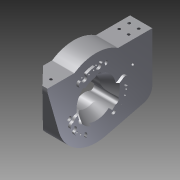
# Autodesk Inventor part: launcher.housing2
Saved by Autodesk Inventor 2011 (Build 150239000, 239)
## iProperties
Created: 2011-01-27
Part Number: launcher.housing2
Document SubType Name: Modeling
Designer: Casey
Density: 1 g/cm^3
Mass: 704.398 g
Surface Area: 699.987 cm^2
Volume: 704.398 cm^3
Author: Casey
Autodesk Inventor part; units mm, degrees
ref_plane "YZ Plane" through (0, 0, 0) normal (1, 0, 0) x (0, 1, 0)
ref_plane "XZ Plane" through (0, 0, 0) normal (0, 1, 0) x (-1, 0, 0)
ref_plane "XY Plane" through (0, 0, 0) normal (0, 0, 1) x (1, 0, 0)
sketch "Sketch1" plane through (0, 0, 0) normal (0, 0, 1) x (1, 0, 0)
  line L0 (2.019581, 25) -> (20, 35.381)
  line L1 (20, 35.381) -> (20, 70)
  line L2 (20, 70) -> (0, 70)
  line L3 (0, 0) -> (46.562095, 0) construction
  line L4 (0, 70) -> (0, 25)
  line L5 (0, 25) -> (2.019581, 25)
  line L6 (0, 25) -> (-20, 25)
  line L7 (-20, 25) -> (-20, 70)
  line L8 (-20, 70) -> (0, 70)
  dimension "d3" = 70
  dimension "d6" = 30
  dimension "d8" = 25
  dimension "d86" = 35.381
  dimension "d182" = 20
  dimension "d230" = 20
  constraints: 18 end point, 2 horizontal, 2 perpendicular, 2 vertical, 1 collinear, 1 parallel, 1 point on line, 1 other
  measures "d3" distance from line of L3.start L2
  measures "d6" angle of L5 L0
  measures "d8" distance from line of L3.start L5
  measures "d86" distance from line of L3 L0.end
  measures "d182" distance between parallel lines of L4 L1
  measures "d230" distance of L4.end L6.end
revolve "Revolution1" add sketch "Sketch1" angle 360 about axis through (0, 0, 0) along (1, 0, 0)
sketch "Sketch11" plane through (20, 0, 0) normal (1, 0, 0) x (0, 0, -1)
  circle A0 centre (0, 0) radius 35.381 projected
  line L0 (-35, -6) -> (0, -6)
  line L1 (0, -6) -> (0, 6)
  line L2 (0, 6) -> (-35, 6)
  arc A1 (-35, 6) -> (-35, -6) centre (-35, 0) ccw
  line L3 (-35, 0) -> (0, 0) construction
  dimension "d87" = 12
  dimension "d88" = 35
  constraints: 8 end point, 2 horizontal, 2 midpoint, 2 point on circle, 1 centre point, 1 parallel, 1 perpendicular, 1 point on line, 1 tangent
  measures "d87" diameter of A1
  measures "d88" distance of A0.centre L3.start
extrude "Extrusion10" cut sketch "Sketch11" against normal through all contours L2 L1 L0 A0 | A0 L0 A1 L2 picked at (-11.774646, -0.669544)
fillet "Fillet12" radius 20 2 edges at (-8.9902, 6, 24.2693) (-8.9902, -6, 24.2693)
pattern_circular "Circular Pattern6" count 3 over 360 about axis through (11.00979, 0, 0) along (1, 0, 0) of "Extrusion10", "Fillet12"
sketch "Sketch26" plane through (20, 0, 0) normal (1, 0, 0) x (0, 0, -1)
  arc A0 (12.208765, 33.207849) -> (12.520317, 33.657942) centre (-4.078625, 44.814783) ccw
  arc A1 (22.888474, 27.671884) -> (12.520317, 33.657942) centre (17.5, 30.310889) ccw
  arc A2 (22.888474, 27.671884) -> (22.654458, 27.177025) centre (40.850053, 18.875199) ccw
  arc A3 (22.654458, -27.177025) -> (22.654458, 27.177025) centre (0, 0) ccw
  arc A4 (22.654458, -27.177025) -> (22.888474, -27.671884) centre (40.850053, -18.875199) ccw
  arc A5 (12.520317, -33.657942) -> (22.888474, -27.671884) centre (17.5, -30.310889) ccw
  arc A6 (12.520317, -33.657942) -> (12.208765, -33.207849) centre (-4.078625, -44.814783) ccw
  arc A7 (-34.863223, -6.030824) -> (12.208765, -33.207849) centre (0, 0) ccw
  arc A8 (-34.863223, -6.030824) -> (-35.408791, -5.986058) centre (-36.771429, -25.939584) ccw
  arc A9 (-35.408791, 5.986058) -> (-35.408791, -5.986058) centre (-35, 0) ccw
  arc A10 (-35.408791, 5.986058) -> (-34.863223, 6.030824) centre (-36.771429, 25.939584) ccw
  arc A11 (12.208765, 33.207849) -> (-34.863223, 6.030824) centre (0, 0) ccw
  circle A12 centre (0, 0) radius 70
  circle A13 centre (0, 0) radius 54.5
  dimension "d183" = 109
  constraints: 1 centre point, 1 coincident
  measures "d183" diameter of A13
extrude "Extrusion14" add sketch "Sketch26" along normal blind 4.5 contours A13
sketch "Sketch27" plane through (0, 0, 0) normal (0, 0, 1) x (1, 0, 0)
  line L0 (20, 35.381) -> (24.5, 37.979076)
  line L1 (24.5, 37.979076) -> (24.5, 35.381)
  line L2 (24.5, 35.381) -> (20, 35.381)
  line L3 (20, 35.381) -> (2.42675, 25.235079)
  line L4 (24.5, 54.5) -> (24.5, -54.5)
  line L5 (0, 0) -> (24.5, 0) construction
  constraints: 8 end point, 2 collinear, 1 midpoint, 1 perpendicular, 1 vertical
revolve "Revolution3" cut sketch "Sketch27" angle 360 about axis through (0, 0, 0) along (1, 0, 0)
sketch "Sketch28" plane through (24.5, 0, 0) normal (1, 0, 0) x (0, 0, -1)
  arc A0 (23.482236, -29.849536) -> (23.482236, 29.849536) centre (0, 0) ccw
  arc A1 (14.109338, 35.260981) -> (-37.591575, 5.411445) centre (0, 0) ccw
  circle A2 centre (0, 0) radius 54.5 construction
  arc A3 (-51.213248, 18.640098) -> (-43.045959, 12.148551) centre (-46.044938, 16.758987) ccw
  circle A4 centre (-46.044938, 16.758987) radius 4 construction
  line L0 (0, 0) -> (-46.044938, 16.758987) construction
  line L1 (0, 0) -> (-54.5, 0) construction
  arc A5 (-35.688658, 12.989609) -> (-43.045959, 12.148551) centre (-38.52465, 5.197784) ccw
  line L2 (0, 0) -> (-27.25, 47.198385) construction
  line L3 (0, 0) -> (-41.749422, 35.031925) construction
  line L4 (0, 0) -> (-9.463826, 53.672023) construction
  arc A6 (-6.594997, 37.402089) -> (-18.086825, 51.411251) centre (-46.044938, 16.758987) ccw
  arc A7 (-18.086825, 51.411251) -> (-51.213248, 18.640098) centre (0, 0) ccw
  line L5 (-35.688658, 12.989609) -> (0, 0)
  line L6 (0, 0) -> (-1.913763, 10.853491)
  arc A8 (-1.913763, 10.853491) -> (-6.594997, 37.402089) centre (-46.044938, 16.758987) ccw
  dimension "d187" = 11
  dimension "d188" = 8
  dimension "d190" = 20
  dimension "d191" = 60
  dimension "d192" = 20
  constraints: 18 point on circle, 14 end point, 6 centre point, 5 point on line, 4 tangent, 3 coincident, 2 collinear, 2 concentric, 1 horizontal, 1 other
  measures "d187" diameter of A3
  measures "d188" diameter of A4
  measures "d190" angle of L1 L0
  measures "d191" angle of L1 L2
  measures "d192" angle of L2 L3
extrude "Extrusion15" cut sketch "Sketch28" against normal up to surface (4.5 mm away)
fillet "Fillet13" radius 6 2 edges at (22.25, 18.6401, 51.2132) (22.25, 51.4113, 18.0868)
sketch "Sketch30" plane through (24.5, 0, 0) normal (1, 0, 0) x (0, 0, -1)
  arc A0 (14.109338, 35.260981) -> (-6.594997, 37.402089) centre (0, 0) ccw
  arc A1 (-54.1534, 6.136711) -> (-7.188402, 54.023855) centre (0, 0) ccw
  circle A2 centre (-51, 0) radius 5
  circle A3 centre (0, 51) radius 5
  line L0 (-51, 0) -> (0, 0) construction
  line L1 (0, 0) -> (0, 51) construction
  dimension "d199" = 51
  dimension "d200" = 10
  dimension "d201" = 90
  constraints: 4 end point, 2 centre point, 1 equal radius, 1 horizontal, 1 perpendicular
  measures "d199" distance of A0.centre L0.start
  measures "d200" diameter of A2
  measures "d201" angle of L0 L1
extrude "Extrusion17" cut sketch "Sketch30" against normal up to surface (4.5 mm away)
sketch "Sketch29" plane through (20, 0, 0) normal (1, 0, 0) x (0, 0, -1)
  arc A0 (-5.412525, 34.96455) -> (-11.105373, 44.357217) centre (-46.044938, 16.758987) ccw
  circle A1 centre (-46.044938, 16.758987) radius 4
  arc A2 (-3.689089, 54.375) -> (3.689089, 54.375) centre (0, 51) ccw
  arc A3 (-54.375, -3.689089) -> (-54.375, 3.689089) centre (-51, 0) ccw
  circle A4 centre (-51, 0) radius 1.5
  circle A5 centre (0, 51) radius 1.5
  dimension "d196" = 8
  dimension "d205" = 3
  constraints: 3 centre point, 3 coincident, 1 equal radius
  measures "d196" diameter of A1
  measures "d205" diameter of A4
extrude "Extrusion16" cut sketch "Sketch29" against normal blind 4
fillet "Fillet14" radius 2 4 edges at (22.25, 54.375, 3.6891) (22.25, 54.375, -3.6891) (22.25, -3.6891, 54.375) (22.25, 3.6891, 54.375)
sketch "Sketch32" plane through (24.5, 0, 0) normal (1, 0, 0) x (0, 0, -1)
  arc A0 (-4.944329, 51.744048) -> (4.944329, 51.744048) centre (0, 51) ccw
  arc A1 (-35.688658, 12.989609) -> (-37.591575, 5.411445) centre (0, 0) ccw
  circle A2 centre (8.769021, 49.731588) radius 1.5
  line L0 (0, 0) -> (8.769021, 49.731588) construction
  line L1 (0, 0) -> (17.271599, 47.453329) construction
  circle A3 centre (17.271599, 47.453329) radius 1.5
  line L2 (0, 0) -> (0, 51) construction
  dimension "d212" = 10
  dimension "d213" = 3
  dimension "d214" = 10
  constraints: 6 end point, 2 centre point, 1 coincident, 1 equal length, 1 equal radius, 1 vertical
  measures "d212" angle of L0 L1
  measures "d213" diameter of A2
  measures "d214" angle of L2 L0
extrude "Extrusion18" cut sketch "Sketch32" against normal blind 6
pattern_circular "Circular Pattern7" count 3 over 360 about axis through (11.00979, 0, 0) along (1, 0, 0) of "Fillet14", "Extrusion16", "Extrusion17", "Fillet13", "Extrusion15", "Extrusion18"
sketch "Sketch42" plane through (20, 0, 0) normal (1, 0, 0) x (0, 0, -1)
  circle A0 centre (0, 0) radius 70
  circle A1 centre (0, 0) radius 70
  line L0 (-58, 101) -> (47, 101)
  line L1 (-70, 0) -> (-70, 42.722229)
  line L2 (0, 0) -> (-15.987577, 0)
  line L3 (47, 101) -> (67.928123, 16.904735)
  line L4 (-58, 101) -> (-58, 39.191836)
  line L5 (-58, -87.65) -> (-52, -87.65)
  line L6 (-58, -87.65) -> (-58, -39.191836)
  line L7 (-52, -87.65) -> (19.223278, -67.308733)
  dimension "d249" = 12
  dimension "d250" = 101
  dimension "d251" = 105
  dimension "d252" = 6
  dimension "d253" = 188.65
  constraints: 16 end point, 8 point on circle, 5 perpendicular, 4 tangent, 1 centre point, 1 coincident, 1 collinear, 1 concentric, 1 horizontal
  measures "d249" distance from line of L1 L0.start
  measures "d250" distance between parallel lines of L2 L0
  measures "d251" distance of L0.start L0.end
  measures "d252" distance of L5.start L5.end
  measures "d253" distance between parallel lines of L5 L0
extrude "Extrusion22" add sketch "Sketch42" against normal up to surface (40 mm away) contours A0 L4 L0 L3 | L7 L5 L6 A0
fillet "Fillet17" radius 20 2 edges at (0, 101, -47) (0, -87.65, 52)
fillet "Fillet18" radius 3 2 edges at (0, -39.1918, 58) (0, 39.1918, 58)
sketch "Sketch43" plane through (20, 101, 58) normal (1, 0, 0) x (0, 0, -1)
  arc A0 (77.223278, -168.308733) -> (125.928123, -84.095265) centre (58, -101) ccw
  line L0 (0, -188.65) -> (3.199992, -188.65)
  arc A1 (108.379214, -121.789054) -> (108.380231, -121.786589) centre (58, -101) ccw
  line L1 (58, -101) -> (58, -87.563984) construction
  line L2 (57.05279, -96.856487) -> (38.730064, -35)
  circle A2 centre (38.730064, -35) radius 2.3815
  dimension "d258" = 16.5
  dimension "d259" = 66
  dimension "d260" = 4.763
  constraints: 4 end point, 1 centre point, 1 coincident, 1 perpendicular
  measures "d258" angle of L1 L2
  measures "d259" vertical distance of A0.centre L2.end
  measures "d260" diameter of A2
extrude "Extrusion23" cut sketch "Sketch43" against normal through all
sketch "Sketch44" plane through (-20, -87.65, 58) normal (0, 0, 1) x (1, 0, 0)
  line L0 (40, 47.550125) -> (40, 0)
  line L1 (20, 87.65) -> (20, -61.026426)
  line L2 (20, -61.026426) -> (20, 235.97281)
  line L3 (28.5, 235.97281) -> (28.5, -61.026426)
  circle A0 centre (28.5, 175.65) radius 3
  circle A1 centre (28.5, 157.65) radius 3
  line L4 (20, 87.65) -> (129.361261, 87.65)
  circle A2 centre (28.5, 17.65) radius 3
  line L5 (20, 175.65) -> (28.5, 175.65)
  line L6 (28.5, 157.65) -> (20, 157.65)
  line L7 (28.5, 17.65) -> (20, 17.65)
  circle A3 centre (11.5, 175.65) radius 3
  circle A4 centre (11.5, 157.65) radius 3
  dimension "d263" = 8.5
  dimension "d264" = 6
  dimension "d265" = 6
  dimension "d266" = 6
  dimension "d267" = 70
  dimension "d268" = 140
  dimension "d269" = 18
  constraints: 14 end point, 6 point on line, 5 centre point, 3 parallel, 3 perpendicular, 2 symmetric about line, 1 collinear, 2 other
  measures "d263" distance between parallel lines of L2 L3
  measures "d264" diameter of A0
  measures "d265" diameter of A1
  measures "d266" diameter of A2
  measures "d267" distance from line of L7.start L4
  measures "d268" distance between parallel lines of L6 L7
  measures "d269" distance between parallel lines of L6 L5
hole "Hole6" at (8.5, 88, 58) at (8.5, 70, 58) at (-8.5, 70, 58) at (-8.5, 88, 58) at (8.5, -70, 58) direction (0, 0, -1) diameter 4.917 depth 8 tip angle 118 thread size "M6x1" class "6H" standard "ANSI Metric M Profile"
sketch "Sketch45" plane through (-20, -87.65, 58) normal (0, 0, 1) x (1, 0, 0)
  line L0 (0, 47.550125) -> (0, 0) construction
  line L1 (40, 0) -> (0, 0) construction
  line L2 (31.010917, 32.197327) -> (6.882491, 32.197252) construction
  line L3 (31.011042, -7.802673) -> (31.011018, -0.024067) construction
  line L4 (6.882491, 32.197252) -> (4.27266, 32.197244) construction
  line L5 (-117.519487, 32.196864) -> (4.27266, 32.197244) construction
  line L6 (31.011018, 0) -> (0, 32.197231) construction
  line L7 (31.011018, 0) -> (0, 32.197231)
  line L8 (0, 32.197231) -> (0, 0)
  line L9 (0, 0) -> (31.011018, 0)
  point P0 (20, 87.65)
  constraints: 8 end point, 4 point on line, 2 collinear, 1 perpendicular, 1 other
extrude "Extrusion24" cut sketch "Sketch45" against normal through all
body "Solid1"
